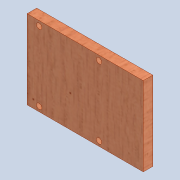
# Autodesk Inventor part: 0005-10-009
Saved by Autodesk Inventor 2020 (Build 240168000, 168)
## iProperties
Created: 2020-12-18
Part Number: 0005-10-009
Material: Generic
Document SubType Name: Modeling
Designer: Iulian Bors
Density: 1 g/cm^3
Appearance: White Oak - Natural Medium Gloss
Author: Iulian Bors
Subject: 009
Autodesk Inventor part; units mm, degrees
ref_plane "YZ Plane" through (0, 0, 0) normal (1, 0, 0) x (0, 1, 0)
ref_plane "XZ Plane" through (0, 0, 0) normal (0, 1, 0) x (-1, 0, 0)
ref_plane "XY Plane" through (0, 0, 0) normal (0, 0, 1) x (1, 0, 0)
sketch "Sketch1" plane through (0, 0, 0) normal (0, 0, 1) x (1, 0, 0)
  line L0 (-48.5, 33) -> (48.5, 33)
  line L1 (48.5, 33) -> (48.5, -33)
  line L2 (48.5, -33) -> (-48.5, -33)
  line L3 (-48.5, -33) -> (-48.5, 33)
  point P0 (0, 0)
  point P1 (0, 33)
  point P2 (-48.5, 0)
  dimension "d0" = 97
  dimension "d1" = 66
  constraints: 8 end point, 2 midpoint, 2 parallel, 1 horizontal, 1 horizontal alignment, 1 perpendicular, 1 vertical alignment
  measures "d0" distance of L0.start L0.end
  measures "d1" distance of L2.end L0.start
extrude "Extrusion1" add sketch "Sketch1" along normal blind 8
sketch "Sketch4" plane through (0, 0, 8) normal (0, 0, 1) x (1, 0, 0)
  line L0 (-48.5, 33) -> (-48.5, -33) projected
  line L1 (-48.5, -33) -> (48.5, -33) projected
  line L2 (48.5, 33) -> (-48.5, 33) projected
  point P0 (0, 0)
  point P1 (-38.5, -29)
  point P2 (-38.5, 29)
  dimension "d19" = 10
  dimension "d20" = 4
  dimension "d21" = 4
  constraints: 1 vertical alignment
  measures "d19" distance from line of point (-38.5, -29) L0
  measures "d20" distance from line of point (-38.5, -29) L1
  measures "d21" distance from line of L2 point (-38.5, 29)
hole "Hole1" at (-38.5, -29, 8) at (-38.5, 29, 8) direction (0, 0, -1) diameter 4.5 end through all
pattern_linear "Rectangular Pattern1" count 2 spacing 50 along (1, 0, 0) of "Hole1"
equation "\"d21\" = d20"
body "Solid1"
